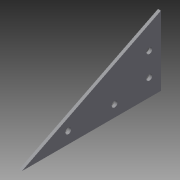
# Autodesk Inventor part: Support_Side_Front
Saved by Autodesk Inventor 2013 (Build 170138000, 138)
## iProperties
Created: 2013-07-13
Part Number: Support_Side_Front
Material: Aluminum 6061
Document SubType Name: Modeling
Designer: orange
Density: 1 g/cm^3
Author: orange
Autodesk Inventor part; units mm, degrees
ref_plane "YZ Plane" through (0, 0, 0) normal (1, 0, 0) x (0, 1, 0)
ref_plane "XZ Plane" through (0, 0, 0) normal (0, 1, 0) x (-1, 0, 0)
ref_plane "XY Plane" through (0, 0, 0) normal (0, 0, 1) x (1, 0, 0)
sketch "Sketch1" plane through (0, 0, 0) normal (1, 0, 0) x (0, 1, 0)
  line L0 (0, 0) -> (0, 152.4)
  line L1 (0, 152.4) -> (76.2, 0)
  line L2 (76.2, 0) -> (0, 0)
  dimension "d0" = 152.4
  dimension "d1" = 76.2
  constraints: 6 end point, 1 perpendicular, 1 vertical
  measures "d0" distance of L0.start L0.end
  measures "d1" distance of L1.end L0.start
extrude "Extrusion1" add sketch "Sketch1" along normal blind 3.175
sketch "Sketch2" plane through (3.175, 0, 0) normal (1, 0, 0) x (0, 0, -1)
  line L0 (-152.4, 0) -> (0, 0) projected
  line L1 (0, 0) -> (0, 76.2) projected
  point P0 (-12.7, 44.45)
  point P1 (-12.7, 19.05)
  dimension "d4" = 12.7
  dimension "d5" = 12.7
  dimension "d6" = 19.05
  dimension "d7" = 25.4
  measures "d4" distance from line of point (-12.7, 44.45) L1
  measures "d5" distance from line of point (-12.7, 19.05) L1
  measures "d6" distance from line of L0 point (-12.7, 19.05)
  measures "d7" distance of point (-12.7, 19.05) point (-12.7, 44.45)
hole "Hole2" at (3.175, 44.45, 12.7) at (3.175, 19.05, 12.7) direction (-1, 0, 0) diameter 6.35 end through all
sketch "Sketch4" plane through (3.175, 0, 0) normal (1, 0, 0) x (0, 0, -1)
  line L0 (-152.4, 0) -> (0, 0) projected
  line L1 (0, 0) -> (0, 76.2) projected
  point P0 (-101.6, 12.7)
  point P1 (-50.8, 12.7)
  dimension "d25" = 12.7
  dimension "d26" = 12.7
  dimension "d27" = 50.8
  dimension "d28" = 50.8
  measures "d25" distance from line of L0 point (-101.6, 12.7)
  measures "d26" distance from line of L0 point (-50.8, 12.7)
  measures "d27" distance from line of point (-50.8, 12.7) L1
  measures "d28" distance of point (-101.6, 12.7) point (-50.8, 12.7)
hole "Hole3" at (3.175, 12.7, 101.6) at (3.175, 12.7, 50.8) direction (-1, 0, 0) diameter 6.35 end through all
body "Solid1"
